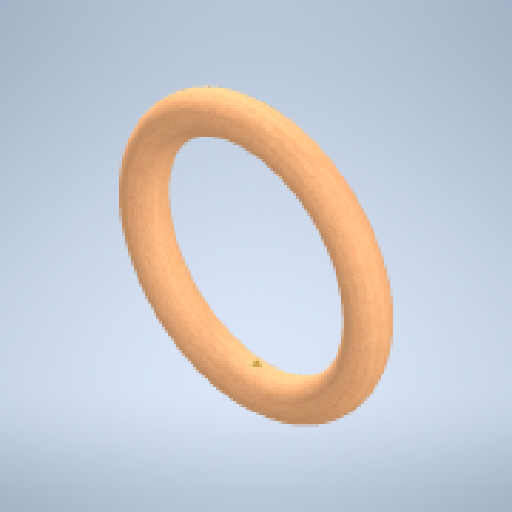
# Autodesk Inventor part: ring
Saved by Autodesk Inventor 2024 (Build 280153000, 153)
## iProperties
Created: 2023-05-23
Part Number: ring
Material: Wood (Cherry)
Document SubType Name: Modeling
Designer: Patrick
Density: 0.63 g/cm^3
Appearance: Cherry - Natural Low Gloss
Author: Patrick
Autodesk Inventor part; units mm, degrees
ref_plane "YZ Plane" through (0, 0, 0) normal (1, 0, 0) x (0, 1, 0)
ref_plane "XZ Plane" through (0, 0, 0) normal (0, 1, 0) x (-1, 0, 0)
ref_plane "XY Plane" through (0, 0, 0) normal (0, 0, 1) x (1, 0, 0)
sketch "Sketch1" plane through (0, 0, 0) normal (1, 0, 0) x (0, 1, 0)
  circle A0 centre (101.5, 0) radius 16
  line L0 (0, 22.4) -> (0, -22.4) projected
  point P0 (0, 0)
  point P1 (117.5, 0)
  dimension "d0" = 32
  dimension "d1" = 235
  constraints: 3 horizontal alignment, 2 other
  measures "d1" diameter of point (117.5, 0) L0
revolve "Revolution1" add sketch "Sketch1" angle 360 about axis through (0, 0, 0) along (0, 0, -1)
ref_plane "Work Plane1" through (0, -85.5, 0) normal (0, 1, 0) x (-1, 0, 0)
body "Solid1"
